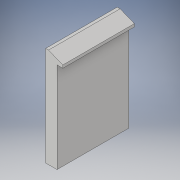
# Autodesk Inventor part: straight
Saved by Autodesk Inventor 2019 (Build 230136000, 136)
## iProperties
Created: 2019-01-18
Part Number: straight
Material: Generic
Document SubType Name: Modeling
Designer: assman
Density: 1 g/cm^3
Appearance: Default
Author: assman
Autodesk Inventor part; units mm, degrees
ref_plane "YZ Plane" through (0, 0, 0) normal (1, 0, 0) x (0, 1, 0)
ref_plane "XZ Plane" through (0, 0, 0) normal (0, 1, 0) x (-1, 0, 0)
ref_plane "XY Plane" through (0, 0, 0) normal (0, 0, 1) x (1, 0, 0)
sketch "Sketch1" plane through (0, 0, 0) normal (0, 1, 0) x (-1, 0, 0)
  line L0 (-0.8, -5) -> (0.8, -5)
  line L1 (0.8, -5) -> (0.8, 5)
  line L2 (0.8, 5) -> (-0.8, 5)
  line L3 (-0.8, 5) -> (-0.8, -5)
  line L4 (-0.8, -5) -> (0.8, 5) construction
  line L5 (0.8, -5) -> (-0.8, 5) construction
  point P0 (0, 0)
  dimension "length" = 10
  dimension "width" = 1.6
  constraints: 12 end point, 2 midpoint, 2 parallel, 1 horizontal, 1 perpendicular
  measures "length" distance of L0.end L1.end
  measures "width" distance of L1.end L2.end
extrude "Extrusion1" add sketch "Sketch1" along normal blind 12.65
sketch "Sketch3" plane through (-0.8, 0, 5) normal (0, 0, 1) x (1, 0, 0)
  line L0 (1.6, 12.65) -> (2.4, 12.65)
  line L1 (1.6, 0) -> (1.6, 12.65)
  line L2 (2.4, 12.65) -> (2.4, 13.05)
  line L3 (0, 13.8434) -> (0.4, 13.8434)
  line L4 (2.4, 13.05) -> (0.4, 13.8434)
  line L5 (0, 0) -> (0, 12.65) projected
  line L6 (0, 0) -> (0, 12.65) projected
  line L7 (0, 13.8434) -> (0, 12.65)
  line L8 (0, 12.65) -> (1.6, 12.65)
  line L9 (1.6, 0) -> (1.6, 12.65) projected
  point P0 (0.8, 0)
  dimension "fixer" = 0.8
  dimension "d8" = 0.4
  dimension "d11" = 0.4
  constraints: 14 end point, 3 perpendicular, 2 collinear
  measures "fixer" distance of L0.start L0.end
  measures "d8" distance of L0.end L2.end
  measures "d11" distance of L3.start L3.end
extrude "Extrusion2" add sketch "Sketch3" against normal blind 10
equation "\"d6\" = length"
equation "\"TOL\" = 0.15"
body "Solid1"
